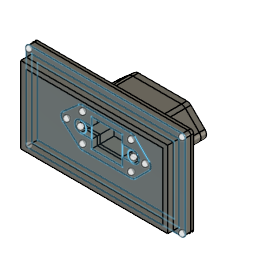
DD-prise-V3 (Autodesk Fusion 360 design; units mm, degrees)
part number: 2025-12-19-16-41-00-752
Autodesk Fusion 360 part; units mm, degrees
sketch "Esquisse1" plane through (0, 0, 0) normal (0, 1, 0) x (1, 0, 0)
  circle A0 centre (-9, 0) radius 2
  circle A1 centre (10, 0) radius 2
  line L0 (15.5858, -1.4142) -> (10.5858, -6.4142)
  line L1 (9.1716, -7) -> (-8.2485, -7)
  line L2 (-9.5655, -6.5052) -> (-15.2798, -1.5052)
  line L3 (-15.2798, 1.5052) -> (-9.5655, 6.5052)
  line L4 (-8.2485, 7) -> (9.1716, 7)
  line L5 (10.5858, 6.4142) -> (15.5858, 1.4142)
  line L6 (-27.5, -16) -> (27.5, -16)
  line L7 (27.5, 16) -> (-27.5, 16)
  line L8 (-28.5, 15) -> (-28.5, -15)
  line L9 (-5, -5) -> (6, -5)
  line L10 (6, -5) -> (6, 5)
  line L11 (6, 5) -> (-5, 5)
  line L12 (-5, 5) -> (-5, -5)
  line L13 (26.25, -13.75) -> (-26.5, -13.75)
  line L14 (-26.5, -13.75) -> (-26.5, 13.75)
  line L15 (-26.5, 13.75) -> (26.25, 13.75)
  line L16 (24.5, -12) -> (-24.5, -12)
  line L17 (-24.5, -12) -> (-24.5, 12)
  line L18 (-24.5, 12) -> (24.5, 12)
  line L19 (24.5, 12) -> (24.5, -12)
  line L20 (26.25, -13.75) -> (26.25, 13.75)
  line L21 (28.5, -15) -> (28.5, 15)
  arc A2 (-15.2798, 1.5052) -> (-15.2798, -1.5052) centre (-13.9628, 0) ccw
  arc A3 (-8.2485, 7) -> (-9.5655, 6.5052) centre (-8.2485, 5) ccw
  arc A4 (10.5858, 6.4142) -> (9.1716, 7) centre (9.1716, 5) ccw
  arc A5 (15.5858, -1.4142) -> (15.5858, 1.4142) centre (14.1716, 0) ccw
  arc A6 (9.1716, -7) -> (10.5858, -6.4142) centre (9.1716, -5) ccw
  arc A7 (-9.5655, -6.5052) -> (-8.2485, -7) centre (-8.2485, -5) ccw
  line L22 (-9, 2) -> (-5, 2)
  line L23 (-9, -2) -> (-5, -2)
  line L24 (10, 2) -> (6, 2)
  line L25 (10, -2) -> (6, -2)
  arc A8 (-27.5, 16) -> (-28.5, 15) centre (-27.5, 15) ccw
  arc A9 (28.5, 15) -> (27.5, 16) centre (27.5, 15) ccw
  arc A10 (27.5, -16) -> (28.5, -15) centre (27.5, -15) ccw
  arc A11 (-28.5, -15) -> (-27.5, -16) centre (-27.5, -15) ccw
  dimension "d24" = 1
  dimension "d25" = 1
  dimension "d26" = 1
  constraint horizontal L1
  constraint parallel L1 L4
  constraint perpendicular L0 L5
  constraint horizontal L6
  constraint horizontal L7
  constraint vertical L8
  constraint horizontal L9
  constraint vertical L10
  constraint horizontal L11
  constraint vertical L12
  constraint horizontal L13
  constraint vertical L14
  constraint horizontal L15
  constraint horizontal L16
  constraint vertical L17
  constraint horizontal L18
  constraint vertical L19
  constraint perpendicular L15 L20
  constraint perpendicular L7 L21
  constraint tangent L2 A2
  constraint tangent L3 A2
  constraint tangent L3 A3
  constraint tangent L4 A3
  constraint equal A2 A3
  constraint tangent L4 A4
  constraint tangent L5 A4
  constraint equal A2 A4
  constraint tangent L0 A5
  constraint tangent L5 A5
  constraint equal A2 A5
  constraint tangent L0 A6
  constraint tangent L1 A6
  constraint equal A2 A6
  constraint tangent L1 A7
  constraint tangent L2 A7
  constraint coincident A0 L22.start
  constraint coincident L12 L22.end
  constraint perpendicular L12 L22
  constraint coincident A0 L23.start
  constraint coincident L12 L23.end
  constraint perpendicular L12 L23
  constraint coincident A1 L24.start
  constraint coincident L10 L24.end
  constraint perpendicular L10 L24
  constraint coincident A1 L25.start
  constraint coincident L10 L25.end
  constraint perpendicular L10 L25
  constraint tangent L7 A8
  constraint tangent L8 A8
  constraint tangent L7 A9
  constraint tangent L21 A9
  constraint tangent L6 A10
  constraint tangent L21 A10
  constraint equal A9 A10
  constraint tangent L6 A11
  constraint tangent L8 A11
  measures "d24" radius of A8
  measures "d25" radius of A9
  measures "d26" radius of A11
extrude "Extrusion1" add sketch "Esquisse1" against normal blind 4 contours L13 L14 L15 L20 makes body 1
extrude "Extrusion2" add sketch "Esquisse1" along normal blind 2 separate body contours L0 L1 L2 L3 L4 L5 A2 A3 A4 A5 A6 A7 | L6 L7 L8 L21 A8 A9 A10 A11 | L13 L14 L15 L20 | L16 L17 L18 L19 makes body 2
extrude "Extrusion3" add sketch "Esquisse1" along normal blind 18 separate body contours L9 L10 L11 L12 | L0 L1 L2 L3 L4 L5 A2 A3 A4 A5 A6 A7 makes body 3
extrude "Extrusion4" add sketch "Esquisse1" against normal blind 4 separate body contours L13 L14 L15 L20 makes body 4
extrude "Extrusion5" add sketch "Esquisse1" along normal blind 2 separate body contours L0 L1 L2 L3 L4 L5 A2 A3 A4 A5 A6 A7 | L6 L7 L8 L21 A8 A9 A10 A11 | L13 L14 L15 L20 | L16 L17 L18 L19 makes body 5
extrude "Extrusion6" add sketch "Esquisse1" along normal blind 2 separate body contours L6 L7 L8 L21 A8 A9 A10 A11 | L13 L14 L15 L20 | L16 L17 L18 L19 makes body 6
extrude "Extrusion7" add sketch "Esquisse1" along normal blind 20 separate body contours L0 L1 L2 L3 L4 L5 A2 A3 A4 A5 A6 A7 makes body 7
extrude "Extrusion8" add sketch "Esquisse1" against normal blind 2 separate body contours L13 L14 L15 L20 makes body 8
extrude "Extrusion9" add sketch "Esquisse1" along normal blind 3 separate body contours L0 L1 L2 L3 L4 L5 A2 A3 A4 A5 A6 A7 | L6 L7 L8 L21 A8 A9 A10 A11 | L13 L14 L15 L20 | L16 L17 L18 L19 makes body 9
extrude "Extrusion10" add sketch "Esquisse1" along normal blind 18 separate body contours L0 L1 L2 L3 L4 L5 A2 A3 A4 A5 A6 A7 makes body 10
extrude "Extrusion11" cut sketch "Esquisse1" along normal blind 8 contours L9 L10 L11 L12 bodies 3
